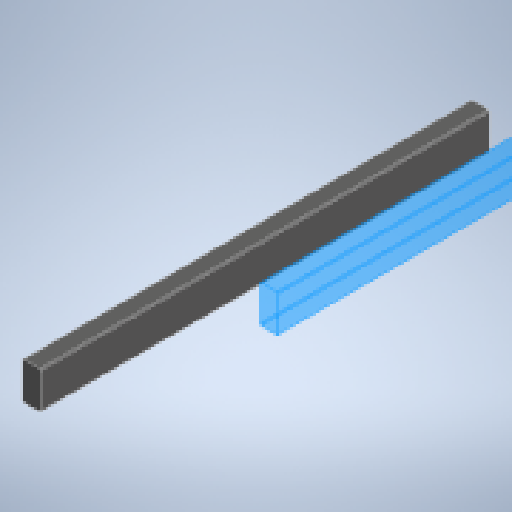
# Autodesk Inventor part: 2x4_Wood
Saved by Autodesk Inventor 2023 (Build 270158000, 158)
## iProperties
Created: 2022-05-10
Part Number: 2x4_Wood
Material: Pine Wood
Document SubType Name: Modeling
Designer: a laptop
Density: 0.498238 g/cm^3
Appearance: Generic
Mass: 3129.97 g
Surface Area: 3752.72 cm^2
Volume: 6282.08 cm^3
Author: a laptop
Autodesk Inventor part; units mm, degrees
ref_plane "YZ Plane" through (0, 0, 0) normal (1, 0, 0) x (0, 1, 0)
ref_plane "XZ Plane" through (0, 0, 0) normal (0, 1, 0) x (-1, 0, 0)
ref_plane "XY Plane" through (0, 0, 0) normal (0, 0, 1) x (1, 0, 0)
sketch "Sketch1" plane through (0, 0, 0) normal (0, 0, 1) x (1, 0, 0)
  line L0 (3.175, 0) -> (47.625, 0)
  line L1 (50.8, 3.175) -> (50.8, 98.425)
  line L2 (47.625, 101.6) -> (3.175, 101.6)
  line L3 (0, 98.425) -> (0, 3.175)
  arc A0 (3.175, 101.6) -> (0, 98.425) centre (3.175, 98.425) ccw
  arc A1 (50.8, 98.425) -> (47.625, 101.6) centre (47.625, 98.425) ccw
  arc A2 (47.625, 0) -> (50.8, 3.175) centre (47.625, 3.175) ccw
  arc A3 (0, 3.175) -> (3.175, 0) centre (3.175, 3.175) ccw
  point P0 (0, 0)
  point P1 (50.8, 101.6)
  point P2 (50.8, 0)
  point P3 (0, 101.6)
  dimension "d0" = 50.8
  dimension "d1" = 101.6
  dimension "d2" = 3.175
  constraints: 8 end point, 8 point on circle, 8 point on line, 8 tangent, 4 centre point, 3 equal radius, 2 parallel, 1 horizontal, 1 perpendicular
  measures "d0" distance of point (50.8, 101.6) point (0, 101.6)
  measures "d1" distance of point (50.8, 0) point (50.8, 101.6)
  measures "d2" radius of A0
extrude "Extrusion1" add sketch "Sketch1" along normal blind 1219.2
body "Solid1"
